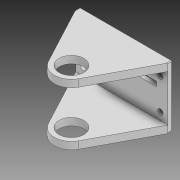
# Autodesk Inventor part: Cablecar_topbracket
Saved by Autodesk Inventor 2020 (Build 240168000, 168)
## iProperties
Created: 2021-02-03
Part Number: Cablecar_topbracket
Material: Generic
Document SubType Name: Modeling
Designer: DDeGo
Density: 1 g/cm^3
Appearance: Default
Author: DDeGo
Autodesk Inventor part; units mm, degrees
ref_plane "YZ Plane" through (0, 0, 0) normal (1, 0, 0) x (0, 1, 0)
ref_plane "XZ Plane" through (0, 0, 0) normal (0, 1, 0) x (-1, 0, 0)
ref_plane "XY Plane" through (0, 0, 0) normal (0, 0, 1) x (1, 0, 0)
sketch "Sketch1" plane through (0, 0, 0) normal (0, 0, 1) x (1, 0, 0)
  line L0 (-29.25, -19.75) -> (29.25, -19.75)
  line L1 (29.75, -19.25) -> (29.75, 19.25)
  line L2 (29.25, 19.75) -> (-29.25, 19.75)
  line L3 (-29.75, 19.25) -> (-29.75, -19.25)
  line L4 (-29.75, -19.75) -> (29.75, 19.75) construction
  line L5 (29.75, -19.75) -> (-29.75, 19.75) construction
  arc A0 (-29.25, 19.75) -> (-29.75, 19.25) centre (-29.25, 19.25) ccw
  arc A1 (29.75, 19.25) -> (29.25, 19.75) centre (29.25, 19.25) ccw
  arc A2 (29.25, -19.75) -> (29.75, -19.25) centre (29.25, -19.25) ccw
  arc A3 (-29.75, -19.25) -> (-29.25, -19.75) centre (-29.25, -19.25) ccw
  line L6 (-25, -10) -> (25, -10) construction
  line L7 (25, -10) -> (25, 10) construction
  line L8 (25, 10) -> (-25, 10) construction
  line L9 (-25, 10) -> (-25, -10) construction
  line L10 (-25, -10) -> (25, 10) construction
  line L11 (25, -10) -> (-25, 10) construction
  circle A4 centre (-25, 10) radius 1.75
  circle A5 centre (-25, -10) radius 1.75
  circle A6 centre (25, -10) radius 1.75
  circle A7 centre (25, 10) radius 1.75
  point P0 (0, 0)
  dimension "d0" = 59.5
  dimension "d1" = 39.5
  dimension "d2" = 0.5
  dimension "d3" = 20
  dimension "d4" = 50
  dimension "d5" = 3.5
  constraints: 24 end point, 8 centre point, 8 point on circle, 8 point on line, 8 tangent, 6 equal radius, 4 coincident, 4 midpoint, 4 parallel, 2 horizontal, 2 perpendicular
  measures "d0" distance of L4.end L5.end
  measures "d1" distance of L5.start L4.end
  measures "d2" radius of A0
  measures "d3" distance of L8.end L6.start
  measures "d4" distance of L7.end L8.end
  measures "d5" diameter of A4
extrude "Extrusion1" add sketch "Sketch1" along normal blind 2.5
sketch "Sketch2" plane through (0, 0, 2.5) normal (0, 0, 1) x (1, 0, 0)
  line L0 (29.75, -19.25) -> (29.75, 19.25) construction
  line L1 (29.75, 15) -> (-29.75, 15)
  line L2 (-29.75, 15) -> (-29.75, 19.25)
  line L3 (29.75, 19.25) -> (29.75, 15)
  line L4 (-29.75, 19.25) -> (-29.75, -19.25) construction
  line L5 (-29.75, -15) -> (29.75, -15)
  line L6 (29.75, -15) -> (29.75, -19.25)
  line L7 (-29.75, -19.25) -> (-29.75, -15)
  line L8 (29.75, -19.25) -> (29.75, 19.25) construction
  line L9 (-29.75, 19.25) -> (-29.75, -19.25) construction
  arc A0 (-29.25, 19.75) -> (-29.75, 19.25) centre (-29.25, 19.25) ccw projected
  line L10 (29.25, 19.75) -> (-29.25, 19.75) projected
  arc A1 (29.75, 19.25) -> (29.25, 19.75) centre (29.25, 19.25) ccw projected
  arc A2 (-29.75, -19.25) -> (-29.25, -19.75) centre (-29.25, -19.25) ccw projected
  line L11 (-29.25, -19.75) -> (29.25, -19.75) projected
  arc A3 (29.25, -19.75) -> (29.75, -19.25) centre (29.25, -19.25) ccw projected
  point P0 (0, 0)
  dimension "d8" = 30
  dimension "d9" = 4.75
  constraints: 12 end point, 4 point on line, 2 horizontal, 2 parallel, 2 perpendicular, 2 tangent, 2 vertical, 1 collinear, 1 point on circle
  measures "d8" distance between parallel lines of L1 L5
  measures "d9" distance between parallel lines of L11 L5
extrude "Extrusion2" add sketch "Sketch2" along normal blind 100
sketch "Sketch3" plane through (-29.25, -19.75, 0) normal (0, -1, 0) x (1, 0, 0)
  line L0 (59, 2.5) -> (59, 102.5) projected
  line L1 (-0.5, 2.5) -> (-0.5, 102.5) projected
  line L2 (-0.5, 2.5) -> (59, 2.5) construction
  line L3 (-0.5, 2.5) -> (59, 2.5) construction
  line L4 (59, 2.5) -> (38.9612, 40.1664)
  line L5 (19.5388, 40.1664) -> (-0.5, 2.5)
  arc A0 (38.9612, 40.1664) -> (19.5388, 40.1664) centre (29.25, 35) ccw
  circle A1 centre (29.25, 35) radius 8
  line L6 (59, 0) -> (59, 102.5) projected
  line L7 (-0.5, 102.5) -> (59, 102.5)
  point P0 (29.25, 0)
  dimension "d13" = 35
  dimension "d14" = 16
  dimension "d15" = 3
  constraints: 8 end point, 2 centre point, 2 point on circle, 2 tangent, 1 coincident, 1 collinear, 1 equal length, 1 horizontal
  measures "d13" distance of point (29.25, 0) A0.centre
  measures "d14" diameter of A1
  measures "d15" radial gap between concentric circles of A0 A1
extrude "Extrusion3" cut sketch "Sketch3" against normal through all
sketch "Sketch4" plane through (0, 0, 2.5) normal (0, 0, 1) x (1, 0, 0)
  line L0 (-22.5, 6) -> (22.5, 6)
  line L1 (22.5, 6) -> (22.5, 3)
  line L2 (22.5, 3) -> (-22.5, 3)
  line L3 (-22.5, 3) -> (-22.5, 6)
  line L4 (-22.5, 6) -> (22.5, 3) construction
  line L5 (22.5, 6) -> (-22.5, 3) construction
  line L6 (0, 4.5) -> (0, 0) construction
  dimension "d18" = 4.5
  dimension "d19" = 3
  dimension "d20" = 45
  constraints: 14 end point, 2 midpoint, 2 parallel, 1 horizontal, 1 perpendicular, 1 vertical
  measures "d18" distance of L6.start L6.end
  measures "d19" distance of L0.end L1.end
  measures "d20" distance of L0.start L0.end
extrude "Extrusion4" cut sketch "Sketch4" against normal through all
body "Solid1"
